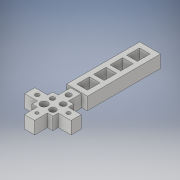
# Autodesk Inventor part: test
Saved by Autodesk Inventor 2019 (Build 230136000, 136)
## iProperties
Created: 2019-02-20
Part Number: test
Material: Generic
Document SubType Name: Modeling
Designer: suchanek
Density: 1 g/cm^3
Appearance: Default
Author: suchanek
Autodesk Inventor part; units mm, degrees
ref_plane "YZ Plane" through (0, 0, 0) normal (1, 0, 0) x (0, 1, 0)
ref_plane "XZ Plane" through (0, 0, 0) normal (0, 1, 0) x (-1, 0, 0)
ref_plane "XY Plane" through (0, 0, 0) normal (0, 0, 1) x (1, 0, 0)
sketch "Sketch1" plane through (0, 0, 0) normal (0, 1, 0) x (-1, 0, 0)
  line L0 (0, 0) -> (10, 0)
  line L1 (10, 0) -> (10, 10)
  line L2 (10, 10) -> (0, 10)
  line L3 (0, 10) -> (0, 0)
  line L4 (0, -6.5) -> (10, -6.5)
  line L5 (10, -6.5) -> (10, -41.5)
  line L6 (10, -41.5) -> (0, -41.5)
  line L7 (0, -41.5) -> (0, -6.5)
  line L8 (2.5, -9) -> (7.5, -9)
  line L9 (7.5, -9) -> (7.5, -15)
  line L10 (7.5, -15) -> (2.5, -15)
  line L11 (2.5, -15) -> (2.5, -9)
  line L12 (2.5, 0) -> (7.5, 0)
  line L13 (7.5, 0) -> (7.5, -6)
  line L14 (7.5, -6) -> (2.5, -6)
  line L15 (2.5, -6) -> (2.5, 0)
  line L16 (10, 7.45) -> (16.05, 7.45)
  line L17 (16.05, 7.45) -> (16.05, 2.5)
  line L18 (16.05, 2.5) -> (10, 2.5)
  line L19 (10, 2.5) -> (10, 7.45)
  line L20 (7.5, 10) -> (2.6, 10)
  line L21 (2.6, 10) -> (2.6, 16.1)
  line L22 (2.6, 16.1) -> (7.5, 16.1)
  line L23 (7.5, 16.1) -> (7.5, 10)
  line L24 (0, 7.45) -> (-6.15, 7.45)
  line L25 (-6.15, 7.45) -> (-6.15, 2.6)
  line L26 (-6.15, 2.6) -> (0, 2.6)
  line L27 (0, 2.6) -> (0, 7.45)
  circle A0 centre (5.1, 12.5) radius 0.75
  circle A1 centre (-2.5, 5) radius 0.9
  circle A2 centre (12.5, 4.95) radius 1
  circle A3 centre (5, -2.5) radius 1.25
  circle A4 centre (2.6, 7.4) radius 1.5
  circle A5 centre (7.1, 7.1) radius 1.75
  circle A6 centre (7.4, 2.8) radius 1.125
  circle A7 centre (2.5, 2.6) radius 1.375
  line L28 (2.5, -24.9) -> (7.5, -24.9)
  line L29 (7.5, -24.9) -> (7.5, -30.85)
  line L30 (7.5, -30.85) -> (2.5, -30.85)
  line L31 (2.5, -30.85) -> (2.5, -24.9)
  line L32 (2.5, -17) -> (7.5, -17)
  line L33 (7.5, -17) -> (7.5, -22.9)
  line L34 (7.5, -22.9) -> (2.5, -22.9)
  line L35 (2.5, -22.9) -> (2.5, -17)
  line L36 (2.5, -32.85) -> (7.5, -32.85)
  line L37 (7.5, -32.85) -> (7.5, -38.9)
  line L38 (7.5, -38.9) -> (2.5, -38.9)
  line L39 (2.5, -38.9) -> (2.5, -32.85)
  dimension "d0" = 10
  dimension "d1" = 10
  dimension "d2" = 10
  dimension "d3" = 35
  dimension "d4" = 5
  dimension "d5" = 6
  dimension "d6" = 2.5
  dimension "d7" = 2.5
  dimension "d8" = 6.5
  dimension "d9" = 5
  dimension "d10" = 6
  dimension "d11" = 6.05
  dimension "d12" = 4.95
  dimension "d13" = 4.9
  dimension "d14" = 6.1
  dimension "d15" = 6.15
  dimension "d16" = 4.85
  dimension "d17" = 2.5
  dimension "d18" = 2.5
  dimension "d19" = 1.5
  dimension "d20" = 1.8
  dimension "d21" = 2
  dimension "d22" = 2.5
  dimension "d23" = 3
  dimension "d24" = 3.5
  dimension "d25" = 2.25
  dimension "d26" = 2.75
  dimension "d27" = 2.5
  dimension "d28" = 2.5
  dimension "d29" = 2.5
  dimension "d30" = 2.5
  dimension "d31" = 2.5
  dimension "d32" = 2.5
  dimension "d33" = 2.4
  dimension "d34" = 2.5
  dimension "d35" = 2.8
  dimension "d36" = 2.5
  dimension "d37" = 2.6
  dimension "d38" = 2.6
  dimension "d39" = 2.6
  dimension "d40" = 2.9
  dimension "d41" = 2.9
  dimension "d42" = 2.6
  dimension "d45" = 5
  dimension "d46" = 5.95
  dimension "d47" = 5
  dimension "d48" = 5.9
  dimension "d49" = 2
  dimension "d50" = 2
  dimension "d51" = 2
  dimension "d52" = 6.05
  constraints: 80 end point, 20 parallel, 10 horizontal, 10 perpendicular, 8 centre point, 7 point on line, 4 collinear
  measures "d0" distance of L2.end L1.end
  measures "d1" distance of L1.end L0.end
  measures "d2" distance of L5.end L6.end
  measures "d3" distance of L4.end L5.end
  measures "d4" distance of L9.end L10.end
  measures "d5" distance of L8.end L9.end
  measures "d6" distance between parallel lines of L4 L8
  measures "d7" distance between parallel lines of L7 L11
  measures "d8" distance between parallel lines of L0 L4
  measures "d9" distance of L13.end L14.end
  measures "d10" distance of L12.end L13.end
  measures "d11" distance of L17.end L18.end
  measures "d12" distance of L16.end L17.end
  measures "d13" distance of L21.end L22.end
  measures "d14" distance of L20.end L21.end
  measures "d15" distance of L26.end L25.end
  measures "d16" distance of L25.end L24.end
  measures "d17" distance between parallel lines of L0 L18
  measures "d18" distance between parallel lines of L1 L13
  measures "d19" diameter of A0
  measures "d20" diameter of A1
  measures "d21" diameter of A2
  measures "d22" diameter of A3
  measures "d23" diameter of A4
  measures "d24" diameter of A5
  measures "d25" diameter of A6
  measures "d26" diameter of A7
  measures "d27" distance from line of L1 A2.centre
  measures "d28" distance from line of L12 A3.centre
  measures "d29" distance from line of L3 A1.centre
  measures "d30" distance from line of L20 A0.centre
  measures "d31" distance from line of L21 A0.centre
  measures "d32" distance from line of L16 A2.centre
  measures "d33" distance from line of A1.centre L26
  measures "d34" distance from line of L15 A3.centre
  measures "d35" distance from line of L0 A6.centre
  measures "d36" distance from line of L3 A7.centre
  measures "d37" distance from line of L0 A7.centre
  measures "d38" distance from line of L27 A4.centre
  measures "d39" distance from line of L2 A4.centre
  measures "d40" distance from line of L20 A5.centre
  measures "d41" distance from line of L1 A5.centre
  measures "d42" distance from line of L1 A6.centre
  measures "d45" distance of L29.end L31.start
  measures "d46" distance of L28.end L29.end
  measures "d47" distance of L33.end L35.start
  measures "d48" distance of L32.end L33.end
  measures "d49" distance between parallel lines of L32 L10
  measures "d50" distance between parallel lines of L34 L28
  measures "d51" distance between parallel lines of L30 L36
  measures "d52" distance of L36.end L37.end
extrude "Extrusion1" add sketch "Sketch1" along normal blind 6
body "Solid1"
